Autodesk Fusion 360 part; units mm, degrees
(part 33 of 40)
  spline S112 degree 5 poles (166.3167, 190.3263) (166.2935, 190.3467) (166.2466, 190.3868) (166.1747, 190.4451) (166.076, 190.5192) (165.9487, 190.6066) (165.8185, 190.6904) (165.6866, 190.772) (165.5538, 190.8524) (165.4203, 190.932) (165.2862, 191.0107) (165.1513, 191.0883) (165.0152, 191.1642) (164.8777, 191.2383) (164.739, 191.3106) (164.5991, 191.3813) (164.4582, 191.4504) (164.3164, 191.5184) (164.1739, 191.5853) (164.0308, 191.6512) (163.887, 191.716) (163.7425, 191.7798) (163.5973, 191.8424) (163.4513, 191.9039) (163.3046, 191.9642) (163.1571, 192.0234) (163.009, 192.0815) (162.8603, 192.1386) (162.711, 192.1947) (162.5611, 192.2499) (162.4106, 192.3041) (162.2596, 192.3574) (162.108, 192.4097) (161.9559, 192.461) (161.8032, 192.5114) (161.65, 192.5608) (161.4962, 192.6094) (161.342, 192.657) (161.1873, 192.7037) (161.0321, 192.7495) (160.8764, 192.7945) (160.7202, 192.8386) (160.5636, 192.8818) (160.4065, 192.9241) (160.249, 192.9656) (160.0911, 193.0063) (159.9327, 193.0461) (159.7739, 193.085) (159.6147, 193.1231) (159.4551, 193.1604) (159.2951, 193.1969) (159.1347, 193.2326) (158.9739, 193.2674) (158.8127, 193.3015) (158.6511, 193.3347) (158.4892, 193.3672) (158.3269, 193.3988) (158.1643, 193.4297) (158.0013, 193.4597) (157.838, 193.489) (157.6743, 193.5175) (157.5103, 193.5453) (157.3459, 193.5723) (157.1812, 193.5984) (157.0162, 193.6239) (156.8509, 193.6486) (156.6853, 193.6725) (156.5194, 193.6956) (156.3531, 193.718) (156.1866, 193.7397) (156.0198, 193.7606) (155.8861, 193.7767) (155.7857, 193.7885) (155.7187, 193.7962) (155.6851, 193.8) knots 0 0 0 0 0 0 0.01428571 0.02857143 0.04285714 0.05714286 0.07142857 0.08571429 0.1 0.11428571 0.12857143 0.14285714 0.15714286 0.17142857 0.18571429 0.2 0.21428571 0.22857143 0.24285714 0.25714286 0.27142857 0.28571429 0.3 0.31428571 0.32857143 0.34285714 0.35714286 0.37142857 0.38571429 0.4 0.41428571 0.42857143 0.44285714 0.45714286 0.47142857 0.48571429 0.5 0.51428571 0.52857143 0.54285714 0.55714286 0.57142857 0.58571429 0.6 0.61428571 0.62857143 0.64285714 0.65714286 0.67142857 0.68571429 0.7 0.71428571 0.72857143 0.74285714 0.75714286 0.77142857 0.78571429 0.8 0.81428571 0.82857143 0.84285714 0.85714286 0.87142857 0.88571429 0.9 0.91428571 0.92857143 0.94285714 0.95714286 0.97142857 0.98571429 1 1 1 1 1 1
  line L8400 (166.3167, 190.3263) -> (166.2935, 190.3467) construction
  line L8401 (166.2935, 190.3467) -> (166.2466, 190.3868) construction
  line L8402 (166.2466, 190.3868) -> (166.1747, 190.4451) construction
  line L8403 (166.1747, 190.4451) -> (166.076, 190.5192) construction
  line L8404 (166.076, 190.5192) -> (165.9487, 190.6066) construction
  line L8405 (165.9487, 190.6066) -> (165.8185, 190.6904) construction
  line L8406 (165.8185, 190.6904) -> (165.6866, 190.772) construction
  line L8407 (165.6866, 190.772) -> (165.5538, 190.8524) construction
  line L8408 (165.5538, 190.8524) -> (165.4203, 190.932) construction
  line L8409 (165.4203, 190.932) -> (165.2862, 191.0107) construction
  line L8410 (165.2862, 191.0107) -> (165.1513, 191.0883) construction
  line L8411 (165.1513, 191.0883) -> (165.0152, 191.1642) construction
  line L8412 (165.0152, 191.1642) -> (164.8777, 191.2383) construction
  line L8413 (164.8777, 191.2383) -> (164.739, 191.3106) construction
  line L8414 (164.739, 191.3106) -> (164.5991, 191.3813) construction
  line L8415 (164.5991, 191.3813) -> (164.4582, 191.4504) construction
  line L8416 (164.4582, 191.4504) -> (164.3164, 191.5184) construction
  line L8417 (164.3164, 191.5184) -> (164.1739, 191.5853) construction
  line L8418 (164.1739, 191.5853) -> (164.0308, 191.6512) construction
  line L8419 (164.0308, 191.6512) -> (163.887, 191.716) construction
  line L8420 (163.887, 191.716) -> (163.7425, 191.7798) construction
  line L8421 (163.7425, 191.7798) -> (163.5973, 191.8424) construction
  line L8422 (163.5973, 191.8424) -> (163.4513, 191.9039) construction
  line L8423 (163.4513, 191.9039) -> (163.3046, 191.9642) construction
  line L8424 (163.3046, 191.9642) -> (163.1571, 192.0234) construction
  line L8425 (163.1571, 192.0234) -> (163.009, 192.0815) construction
  line L8426 (163.009, 192.0815) -> (162.8603, 192.1386) construction
  line L8427 (162.8603, 192.1386) -> (162.711, 192.1947) construction
  line L8428 (162.711, 192.1947) -> (162.5611, 192.2499) construction
  line L8429 (162.5611, 192.2499) -> (162.4106, 192.3041) construction
  line L8430 (162.4106, 192.3041) -> (162.2596, 192.3574) construction
  line L8431 (162.2596, 192.3574) -> (162.108, 192.4097) construction
  line L8432 (162.108, 192.4097) -> (161.9559, 192.461) construction
  line L8433 (161.9559, 192.461) -> (161.8032, 192.5114) construction
  line L8434 (161.8032, 192.5114) -> (161.65, 192.5608) construction
  line L8435 (161.65, 192.5608) -> (161.4962, 192.6094) construction
  line L8436 (161.4962, 192.6094) -> (161.342, 192.657) construction
  line L8437 (161.342, 192.657) -> (161.1873, 192.7037) construction
  line L8438 (161.1873, 192.7037) -> (161.0321, 192.7495) construction
  line L8439 (161.0321, 192.7495) -> (160.8764, 192.7945) construction
  line L8440 (160.8764, 192.7945) -> (160.7202, 192.8386) construction
  line L8441 (160.7202, 192.8386) -> (160.5636, 192.8818) construction
  line L8442 (160.5636, 192.8818) -> (160.4065, 192.9241) construction
  line L8443 (160.4065, 192.9241) -> (160.249, 192.9656) construction
  line L8444 (160.249, 192.9656) -> (160.0911, 193.0063) construction
  line L8445 (160.0911, 193.0063) -> (159.9327, 193.0461) construction
  line L8446 (159.9327, 193.0461) -> (159.7739, 193.085) construction
  line L8447 (159.7739, 193.085) -> (159.6147, 193.1231) construction
  line L8448 (159.6147, 193.1231) -> (159.4551, 193.1604) construction
  line L8449 (159.4551, 193.1604) -> (159.2951, 193.1969) construction
  line L8450 (159.2951, 193.1969) -> (159.1347, 193.2326) construction
  line L8451 (159.1347, 193.2326) -> (158.9739, 193.2674) construction
  line L8452 (158.9739, 193.2674) -> (158.8127, 193.3015) construction
  line L8453 (158.8127, 193.3015) -> (158.6511, 193.3347) construction
  line L8454 (158.6511, 193.3347) -> (158.4892, 193.3672) construction
  line L8455 (158.4892, 193.3672) -> (158.3269, 193.3988) construction
  line L8456 (158.3269, 193.3988) -> (158.1643, 193.4297) construction
  line L8457 (158.1643, 193.4297) -> (158.0013, 193.4597) construction
  line L8458 (158.0013, 193.4597) -> (157.838, 193.489) construction
  line L8459 (157.838, 193.489) -> (157.6743, 193.5175) construction
  line L8460 (157.6743, 193.5175) -> (157.5103, 193.5453) construction
  line L8461 (157.5103, 193.5453) -> (157.3459, 193.5723) construction
  line L8462 (157.3459, 193.5723) -> (157.1812, 193.5984) construction
  line L8463 (157.1812, 193.5984) -> (157.0162, 193.6239) construction
  line L8464 (157.0162, 193.6239) -> (156.8509, 193.6486) construction
  line L8465 (156.8509, 193.6486) -> (156.6853, 193.6725) construction
  line L8466 (156.6853, 193.6725) -> (156.5194, 193.6956) construction
  line L8467 (156.5194, 193.6956) -> (156.3531, 193.718) construction
  line L8468 (156.3531, 193.718) -> (156.1866, 193.7397) construction
  line L8469 (156.1866, 193.7397) -> (156.0198, 193.7606) construction
  line L8470 (156.0198, 193.7606) -> (155.8861, 193.7767) construction
  line L8471 (155.8861, 193.7767) -> (155.7857, 193.7885) construction
  line L8472 (155.7857, 193.7885) -> (155.7187, 193.7962) construction
  line L8473 (155.7187, 193.7962) -> (155.6851, 193.8) construction
  arc A209 (172.7536, 191.8132) -> (172.8837, 194.5906) centre (171.3824, 193.2692) ccw
  arc A210 (214.3883, 221.4115) -> (209.8757, 221.4115) centre (212.132, 150) ccw
  spline S113 degree 5 poles (166.3167, 109.6737) (166.2935, 109.6533) (166.2466, 109.6132) (166.1747, 109.5549) (166.076, 109.4808) (165.9487, 109.3934) (165.8185, 109.3096) (165.6866, 109.228) (165.5538, 109.1476) (165.4203, 109.068) (165.2862, 108.9893) (165.1513, 108.9117) (165.0152, 108.8358) (164.8777, 108.7617) (164.739, 108.6894) (164.5991, 108.6187) (164.4582, 108.5496) (164.3164, 108.4816) (164.1739, 108.4147) (164.0308, 108.3488) (163.887, 108.284) (163.7425, 108.2202) (163.5973, 108.1576) (163.4513, 108.0961) (163.3046, 108.0358) (163.1571, 107.9766) (163.009, 107.9185) (162.8603, 107.8614) (162.711, 107.8053) (162.5611, 107.7501) (162.4106, 107.6959) (162.2596, 107.6426) (162.108, 107.5903) (161.9559, 107.539) (161.8032, 107.4886) (161.65, 107.4392) (161.4962, 107.3906) (161.342, 107.343) (161.1873, 107.2963) (161.0321, 107.2505) (160.8764, 107.2055) (160.7202, 107.1614) (160.5636, 107.1182) (160.4065, 107.0759) (160.249, 107.0344) (160.0911, 106.9937) (159.9327, 106.9539) (159.7739, 106.915) (159.6147, 106.8769) (159.4551, 106.8396) (159.2951, 106.8031) (159.1347, 106.7674) (158.9739, 106.7326) (158.8127, 106.6985) (158.6511, 106.6653) (158.4892, 106.6328) (158.3269, 106.6012) (158.1643, 106.5703) (158.0013, 106.5403) (157.838, 106.511) (157.6743, 106.4825) (157.5103, 106.4547) (157.3459, 106.4277) (157.1812, 106.4016) (157.0162, 106.3761) (156.8509, 106.3514) (156.6853, 106.3275) (156.5194, 106.3044) (156.3531, 106.282) (156.1866, 106.2603) (156.0198, 106.2394) (155.8861, 106.2233) (155.7857, 106.2115) (155.7187, 106.2038) (155.6851, 106.2) knots 0 0 0 0 0 0 0.01428571 0.02857143 0.04285714 0.05714286 0.07142857 0.08571429 0.1 0.11428571 0.12857143 0.14285714 0.15714286 0.17142857 0.18571429 0.2 0.21428571 0.22857143 0.24285714 0.25714286 0.27142857 0.28571429 0.3 0.31428571 0.32857143 0.34285714 0.35714286 0.37142857 0.38571429 0.4 0.41428571 0.42857143 0.44285714 0.45714286 0.47142857 0.48571429 0.5 0.51428571 0.52857143 0.54285714 0.55714286 0.57142857 0.58571429 0.6 0.61428571 0.62857143 0.64285714 0.65714286 0.67142857 0.68571429 0.7 0.71428571 0.72857143 0.74285714 0.75714286 0.77142857 0.78571429 0.8 0.81428571 0.82857143 0.84285714 0.85714286 0.87142857 0.88571429 0.9 0.91428571 0.92857143 0.94285714 0.95714286 0.97142857 0.98571429 1 1 1 1 1 1
  line L8474 (166.3167, 109.6737) -> (166.2935, 109.6533) construction
  line L8475 (166.2935, 109.6533) -> (166.2466, 109.6132) construction
  line L8476 (166.2466, 109.6132) -> (166.1747, 109.5549) construction
  line L8477 (166.1747, 109.5549) -> (166.076, 109.4808) construction
  line L8478 (166.076, 109.4808) -> (165.9487, 109.3934) construction
  line L8479 (165.9487, 109.3934) -> (165.8185, 109.3096) construction
  line L8480 (165.8185, 109.3096) -> (165.6866, 109.228) construction
  line L8481 (165.6866, 109.228) -> (165.5538, 109.1476) construction
  line L8482 (165.5538, 109.1476) -> (165.4203, 109.068) construction
  line L8483 (165.4203, 109.068) -> (165.2862, 108.9893) construction
  line L8484 (165.2862, 108.9893) -> (165.1513, 108.9117) construction
  line L8485 (165.1513, 108.9117) -> (165.0152, 108.8358) construction
  line L8486 (165.0152, 108.8358) -> (164.8777, 108.7617) construction
  line L8487 (164.8777, 108.7617) -> (164.739, 108.6894) construction
  line L8488 (164.739, 108.6894) -> (164.5991, 108.6187) construction
  line L8489 (164.5991, 108.6187) -> (164.4582, 108.5496) construction
  line L8490 (164.4582, 108.5496) -> (164.3164, 108.4816) construction
  line L8491 (164.3164, 108.4816) -> (164.1739, 108.4147) construction
  line L8492 (164.1739, 108.4147) -> (164.0308, 108.3488) construction
  line L8493 (164.0308, 108.3488) -> (163.887, 108.284) construction
  line L8494 (163.887, 108.284) -> (163.7425, 108.2202) construction
  line L8495 (163.7425, 108.2202) -> (163.5973, 108.1576) construction
  line L8496 (163.5973, 108.1576) -> (163.4513, 108.0961) construction
  line L8497 (163.4513, 108.0961) -> (163.3046, 108.0358) construction
  line L8498 (163.3046, 108.0358) -> (163.1571, 107.9766) construction
  line L8499 (163.1571, 107.9766) -> (163.009, 107.9185) construction
  line L8500 (163.009, 107.9185) -> (162.8603, 107.8614) construction
  line L8501 (162.8603, 107.8614) -> (162.711, 107.8053) construction
  line L8502 (162.711, 107.8053) -> (162.5611, 107.7501) construction
  line L8503 (162.5611, 107.7501) -> (162.4106, 107.6959) construction
  line L8504 (162.4106, 107.6959) -> (162.2596, 107.6426) construction
  line L8505 (162.2596, 107.6426) -> (162.108, 107.5903) construction
  line L8506 (162.108, 107.5903) -> (161.9559, 107.539) construction
  line L8507 (161.9559, 107.539) -> (161.8032, 107.4886) construction
  line L8508 (161.8032, 107.4886) -> (161.65, 107.4392) construction
  line L8509 (161.65, 107.4392) -> (161.4962, 107.3906) construction
  line L8510 (161.4962, 107.3906) -> (161.342, 107.343) construction
  line L8511 (161.342, 107.343) -> (161.1873, 107.2963) construction
  line L8512 (161.1873, 107.2963) -> (161.0321, 107.2505) construction
  line L8513 (161.0321, 107.2505) -> (160.8764, 107.2055) construction
  line L8514 (160.8764, 107.2055) -> (160.7202, 107.1614) construction
  line L8515 (160.7202, 107.1614) -> (160.5636, 107.1182) construction
  line L8516 (160.5636, 107.1182) -> (160.4065, 107.0759) construction
  line L8517 (160.4065, 107.0759) -> (160.249, 107.0344) construction
  line L8518 (160.249, 107.0344) -> (160.0911, 106.9937) construction
  line L8519 (160.0911, 106.9937) -> (159.9327, 106.9539) construction
  line L8520 (159.9327, 106.9539) -> (159.7739, 106.915) construction
  line L8521 (159.7739, 106.915) -> (159.6147, 106.8769) construction
  line L8522 (159.6147, 106.8769) -> (159.4551, 106.8396) construction
  line L8523 (159.4551, 106.8396) -> (159.2951, 106.8031) construction
  line L8524 (159.2951, 106.8031) -> (159.1347, 106.7674) construction
  line L8525 (159.1347, 106.7674) -> (158.9739, 106.7326) construction
  line L8526 (158.9739, 106.7326) -> (158.8127, 106.6985) construction
  line L8527 (158.8127, 106.6985) -> (158.6511, 106.6653) construction
  line L8528 (158.6511, 106.6653) -> (158.4892, 106.6328) construction
  line L8529 (158.4892, 106.6328) -> (158.3269, 106.6012) construction
  line L8530 (158.3269, 106.6012) -> (158.1643, 106.5703) construction
  line L8531 (158.1643, 106.5703) -> (158.0013, 106.5403) construction
  line L8532 (158.0013, 106.5403) -> (157.838, 106.511) construction
  line L8533 (157.838, 106.511) -> (157.6743, 106.4825) construction
  line L8534 (157.6743, 106.4825) -> (157.5103, 106.4547) construction
  line L8535 (157.5103, 106.4547) -> (157.3459, 106.4277) construction
  line L8536 (157.3459, 106.4277) -> (157.1812, 106.4016) construction
  line L8537 (157.1812, 106.4016) -> (157.0162, 106.3761) construction
  line L8538 (157.0162, 106.3761) -> (156.8509, 106.3514) construction
  line L8539 (156.8509, 106.3514) -> (156.6853, 106.3275) construction
  line L8540 (156.6853, 106.3275) -> (156.5194, 106.3044) construction
  line L8541 (156.5194, 106.3044) -> (156.3531, 106.282) construction
  line L8542 (156.3531, 106.282) -> (156.1866, 106.2603) construction
  line L8543 (156.1866, 106.2603) -> (156.0198, 106.2394) construction
  line L8544 (156.0198, 106.2394) -> (155.8861, 106.2233) construction
  line L8545 (155.8861, 106.2233) -> (155.7857, 106.2115) construction
  line L8546 (155.7857, 106.2115) -> (155.7187, 106.2038) construction
  line L8547 (155.7187, 106.2038) -> (155.6851, 106.2) construction
  arc A211 (187.9188, 82.7809) -> (192.2105, 81.3864) centre (212.132, 150) ccw
  arc A212 (251.5104, 108.1868) -> (253.9452, 110.6216) centre (212.132, 150) ccw
  arc A213 (262.5041, 122.4018) -> (264.0674, 125.4699) centre (212.132, 150) ccw
  line L8548 (172.8837, 105.4094) -> (171.8057, 104.1847)
  line L8549 (199.127, 92.0377) -> (198.7698, 90.4458)
  line L8550 (235.6801, 95.4634) -> (236.3268, 93.9655)
  line L8551 (225.137, 92.0377) -> (225.4942, 90.4458)
  arc A214 (253.9452, 189.3784) -> (256.7226, 189.2483) centre (255.4012, 190.7496) ccw
  arc A215 (217.6748, 209.1442) -> (219.4126, 206.9737) centre (219.6661, 208.9575) ccw
  line L8552 (256.7226, 189.2483) -> (257.9473, 190.3263)
  line L8553 (161.0254, 119.7202) -> (159.6217, 118.8885)
  line L8554 (256.7226, 189.2483) -> (257.9473, 190.3263)
  line L8555 (270.0943, 163.005) -> (271.6862, 163.3622)
  line L8556 (271.2762, 144.4572) -> (272.9005, 144.3049)
  line L8557 (167.5414, 110.7517) -> (166.3167, 109.6737)
  arc A216 (252.2812, 90.9007) -> (255.932, 93.5531) centre (212.132, 150) ccw
  spline S114 degree 5 poles (268.1665, 174.1948) (268.1948, 174.2071) (268.2518, 174.2308) (268.3382, 174.264) (268.4549, 174.3039) (268.6031, 174.3478) (268.7528, 174.3873) (268.9034, 174.4241) (269.0546, 174.4595) (269.2061, 174.494) (269.358, 174.5274) (269.5103, 174.5594) (269.6632, 174.5896) (269.8168, 174.6176) (269.9711, 174.6435) (270.126, 174.6674) (270.2814, 174.6897) (270.4372, 174.7105) (270.5934, 174.7301) (270.7499, 174.7485) (270.9067, 174.7658) (271.0638, 174.7818) (271.2213, 174.7965) (271.3791, 174.8098) (271.5373, 174.8218) (271.6958, 174.8325) (271.8546, 174.842) (272.0137, 174.8504) (272.1731, 174.8577) (272.3327, 174.8638) (272.4925, 174.8689) (272.6526, 174.8729) (272.8129, 174.8757) (272.9735, 174.8776) (273.1343, 174.8783) (273.2953, 174.878) (273.4565, 174.8766) (273.6179, 174.8742) (273.7795, 174.8708) (273.9413, 174.8665) (274.1032, 174.8611) (274.2654, 174.8548) (274.4277, 174.8475) (274.5901, 174.8392) (274.7527, 174.83) (274.9155, 174.8199) (275.0784, 174.8088) (275.2415, 174.7967) (275.4047, 174.7838) (275.568, 174.77) (275.7315, 174.7552) (275.8951, 174.7396) (276.0588, 174.723) (276.2226, 174.7056) (276.3865, 174.6873) (276.5505, 174.6681) (276.7146, 174.648) (276.8788, 174.6271) (277.0431, 174.6054) (277.2075, 174.5828) (277.372, 174.5593) (277.5366, 174.535) (277.7012, 174.5098) (277.866, 174.4839) (278.0307, 174.4571) (278.1956, 174.4294) (278.3605, 174.401) (278.5255, 174.3718) (278.6905, 174.3417) (278.8556, 174.3108) (279.0207, 174.2792) (279.1528, 174.2532) (279.2519, 174.2334) (279.318, 174.22) (279.3511, 174.2132) knots 0 0 0 0 0 0 0.01428571 0.02857143 0.04285714 0.05714286 0.07142857 0.08571429 0.1 0.11428571 0.12857143 0.14285714 0.15714286 0.17142857 0.18571429 0.2 0.21428571 0.22857143 0.24285714 0.25714286 0.27142857 0.28571429 0.3 0.31428571 0.32857143 0.34285714 0.35714286 0.37142857 0.38571429 0.4 0.41428571 0.42857143 0.44285714 0.45714286 0.47142857 0.48571429 0.5 0.51428571 0.52857143 0.54285714 0.55714286 0.57142857 0.58571429 0.6 0.61428571 0.62857143 0.64285714 0.65714286 0.67142857 0.68571429 0.7 0.71428571 0.72857143 0.74285714 0.75714286 0.77142857 0.78571429 0.8 0.81428571 0.82857143 0.84285714 0.85714286 0.87142857 0.88571429 0.9 0.91428571 0.92857143 0.94285714 0.95714286 0.97142857 0.98571429 1 1 1 1 1 1
  line L8558 (268.1665, 174.1948) -> (268.1948, 174.2071) construction
  line L8559 (268.1948, 174.2071) -> (268.2518, 174.2308) construction
  line L8560 (268.2518, 174.2308) -> (268.3382, 174.264) construction
  line L8561 (268.3382, 174.264) -> (268.4549, 174.3039) construction
  line L8562 (268.4549, 174.3039) -> (268.6031, 174.3478) construction
  line L8563 (268.6031, 174.3478) -> (268.7528, 174.3873) construction
  line L8564 (268.7528, 174.3873) -> (268.9034, 174.4241) construction
  line L8565 (268.9034, 174.4241) -> (269.0546, 174.4595) construction
  line L8566 (269.0546, 174.4595) -> (269.2061, 174.494) construction
  line L8567 (269.2061, 174.494) -> (269.358, 174.5274) construction
  line L8568 (269.358, 174.5274) -> (269.5103, 174.5594) construction
  line L8569 (269.5103, 174.5594) -> (269.6632, 174.5896) construction
  line L8570 (269.6632, 174.5896) -> (269.8168, 174.6176) construction
  line L8571 (269.8168, 174.6176) -> (269.9711, 174.6435) construction
  line L8572 (269.9711, 174.6435) -> (270.126, 174.6674) construction
  line L8573 (270.126, 174.6674) -> (270.2814, 174.6897) construction
  line L8574 (270.2814, 174.6897) -> (270.4372, 174.7105) construction
  line L8575 (270.4372, 174.7105) -> (270.5934, 174.7301) construction
  line L8576 (270.5934, 174.7301) -> (270.7499, 174.7485) construction
  line L8577 (270.7499, 174.7485) -> (270.9067, 174.7658) construction
  line L8578 (270.9067, 174.7658) -> (271.0638, 174.7818) construction
  line L8579 (271.0638, 174.7818) -> (271.2213, 174.7965) construction
  line L8580 (271.2213, 174.7965) -> (271.3791, 174.8098) construction
  line L8581 (271.3791, 174.8098) -> (271.5373, 174.8218) construction
  line L8582 (271.5373, 174.8218) -> (271.6958, 174.8325) construction
  line L8583 (271.6958, 174.8325) -> (271.8546, 174.842) construction
  line L8584 (271.8546, 174.842) -> (272.0137, 174.8504) construction
  line L8585 (272.0137, 174.8504) -> (272.1731, 174.8577) construction
  line L8586 (272.1731, 174.8577) -> (272.3327, 174.8638) construction
  line L8587 (272.3327, 174.8638) -> (272.4925, 174.8689) construction
  line L8588 (272.4925, 174.8689) -> (272.6526, 174.8729) construction
  line L8589 (272.6526, 174.8729) -> (272.8129, 174.8757) construction
  line L8590 (272.8129, 174.8757) -> (272.9735, 174.8776) construction
  line L8591 (272.9735, 174.8776) -> (273.1343, 174.8783) construction
  line L8592 (273.1343, 174.8783) -> (273.2953, 174.878) construction
  line L8593 (273.2953, 174.878) -> (273.4565, 174.8766) construction
  line L8594 (273.4565, 174.8766) -> (273.6179, 174.8742) construction
  line L8595 (273.6179, 174.8742) -> (273.7795, 174.8708) construction
  line L8596 (273.7795, 174.8708) -> (273.9413, 174.8665) construction
  line L8597 (273.9413, 174.8665) -> (274.1032, 174.8611) construction
  line L8598 (274.1032, 174.8611) -> (274.2654, 174.8548) construction
  line L8599 (274.2654, 174.8548) -> (274.4277, 174.8475) construction
  line L8600 (274.4277, 174.8475) -> (274.5901, 174.8392) construction
  line L8601 (274.5901, 174.8392) -> (274.7527, 174.83) construction
  line L8602 (274.7527, 174.83) -> (274.9155, 174.8199) construction
  line L8603 (274.9155, 174.8199) -> (275.0784, 174.8088) construction
  line L8604 (275.0784, 174.8088) -> (275.2415, 174.7967) construction
  line L8605 (275.2415, 174.7967) -> (275.4047, 174.7838) construction
  line L8606 (275.4047, 174.7838) -> (275.568, 174.77) construction
  line L8607 (275.568, 174.77) -> (275.7315, 174.7552) construction
  line L8608 (275.7315, 174.7552) -> (275.8951, 174.7396) construction
  line L8609 (275.8951, 174.7396) -> (276.0588, 174.723) construction
  line L8610 (276.0588, 174.723) -> (276.2226, 174.7056) construction
  line L8611 (276.2226, 174.7056) -> (276.3865, 174.6873) construction
  line L8612 (276.3865, 174.6873) -> (276.5505, 174.6681) construction
  line L8613 (276.5505, 174.6681) -> (276.7146, 174.648) construction
  line L8614 (276.7146, 174.648) -> (276.8788, 174.6271) construction
  line L8615 (276.8788, 174.6271) -> (277.0431, 174.6054) construction
  line L8616 (277.0431, 174.6054) -> (277.2075, 174.5828) construction
  line L8617 (277.2075, 174.5828) -> (277.372, 174.5593) construction
  line L8618 (277.372, 174.5593) -> (277.5366, 174.535) construction
  line L8619 (277.5366, 174.535) -> (277.7012, 174.5098) construction
  line L8620 (277.7012, 174.5098) -> (277.866, 174.4839) construction
  line L8621 (277.866, 174.4839) -> (278.0307, 174.4571) construction
  line L8622 (278.0307, 174.4571) -> (278.1956, 174.4294) construction
  line L8623 (278.1956, 174.4294) -> (278.3605, 174.401) construction
  line L8624 (278.3605, 174.401) -> (278.5255, 174.3718) construction
  line L8625 (278.5255, 174.3718) -> (278.6905, 174.3417) construction
  line L8626 (278.6905, 174.3417) -> (278.8556, 174.3108) construction
  line L8627 (278.8556, 174.3108) -> (279.0207, 174.2792) construction
  line L8628 (279.0207, 174.2792) -> (279.1528, 174.2532) construction
  line L8629 (279.1528, 174.2532) -> (279.2519, 174.2334) construction
  line L8630 (279.2519, 174.2334) -> (279.318, 174.22) construction
  line L8631 (279.318, 174.22) -> (279.3511, 174.2132) construction
  arc A217 (209.8757, 78.5885) -> (214.3883, 78.5885) centre (212.132, 150) ccw
  spline S115 degree 5 poles (198.7698, 209.5542) (198.763, 209.5843) (198.7487, 209.6444) (198.7249, 209.7338) (198.6885, 209.8517) (198.6369, 209.9973) (198.5809, 210.1416) (198.5221, 210.2852) (198.4619, 210.4283) (198.4007, 210.5711) (198.3385, 210.7136) (198.2749, 210.8557) (198.2094, 210.9971) (198.1418, 211.1379) (198.072, 211.2779) (198.0004, 211.4173) (197.927, 211.5561) (197.8523, 211.6944) (197.7763, 211.8322) (197.6993, 211.9697) (197.6211, 212.1067) (197.5416, 212.2432) (197.4609, 212.3792) (197.379, 212.5148) (197.2957, 212.6498) (197.2112, 212.7843) (197.1256, 212.9184) (197.0388, 213.052) (196.951, 213.1852) (196.8622, 213.318) (196.7723, 213.4503) (196.6814, 213.5821) (196.5895, 213.7135) (196.4966, 213.8445) (196.4027, 213.975) (196.3078, 214.105) (196.212, 214.2346) (196.1152, 214.3638) (196.0174, 214.4926) (195.9188, 214.6209) (195.8193, 214.7488) (195.7189, 214.8762) (195.6176, 215.0032) (195.5154, 215.1298) (195.4124, 215.256) (195.3085, 215.3817) (195.2037, 215.507) (195.0982, 215.6318) (194.9918, 215.7562) (194.8846, 215.8802) (194.7765, 216.0038) (194.6677, 216.1269) (194.5581, 216.2497) (194.4478, 216.3719) (194.3366, 216.4938) (194.2247, 216.6152) (194.112, 216.7362) (193.9985, 216.8568) (193.8843, 216.9769) (193.7694, 217.0966) (193.6538, 217.2159) (193.5374, 217.3347) (193.4202, 217.4531) (193.3024, 217.5711) (193.1839, 217.6887) (193.0646, 217.8058) (192.9447, 217.9225) (192.8241, 218.0388) (192.7027, 218.1546) (192.5808, 218.27) (192.4581, 218.385) (192.3594, 218.4767) (192.2851, 218.5452) (192.2354, 218.5908) (192.2105, 218.6136) knots 0 0 0 0 0 0 0.01428571 0.02857143 0.04285714 0.05714286 0.07142857 0.08571429 0.1 0.11428571 0.12857143 0.14285714 0.15714286 0.17142857 0.18571429 0.2 0.21428571 0.22857143 0.24285714 0.25714286 0.27142857 0.28571429 0.3 0.31428571 0.32857143 0.34285714 0.35714286 0.37142857 0.38571429 0.4 0.41428571 0.42857143 0.44285714 0.45714286 0.47142857 0.48571429 0.5 0.51428571 0.52857143 0.54285714 0.55714286 0.57142857 0.58571429 0.6 0.61428571 0.62857143 0.64285714 0.65714286 0.67142857 0.68571429 0.7 0.71428571 0.72857143 0.74285714 0.75714286 0.77142857 0.78571429 0.8 0.81428571 0.82857143 0.84285714 0.85714286 0.87142857 0.88571429 0.9 0.91428571 0.92857143 0.94285714 0.95714286 0.97142857 0.98571429 1 1 1 1 1 1
  line L8632 (198.7698, 209.5542) -> (198.763, 209.5843) construction
  line L8633 (198.763, 209.5843) -> (198.7487, 209.6444) construction
  line L8634 (198.7487, 209.6444) -> (198.7249, 209.7338) construction
  line L8635 (198.7249, 209.7338) -> (198.6885, 209.8517) construction
  line L8636 (198.6885, 209.8517) -> (198.6369, 209.9973) construction
  line L8637 (198.6369, 209.9973) -> (198.5809, 210.1416) construction
  line L8638 (198.5809, 210.1416) -> (198.5221, 210.2852) construction
  line L8639 (198.5221, 210.2852) -> (198.4619, 210.4283) construction
  line L8640 (198.4619, 210.4283) -> (198.4007, 210.5711) construction
  line L8641 (198.4007, 210.5711) -> (198.3385, 210.7136) construction
  line L8642 (198.3385, 210.7136) -> (198.2749, 210.8557) construction
  line L8643 (198.2749, 210.8557) -> (198.2094, 210.9971) construction
  line L8644 (198.2094, 210.9971) -> (198.1418, 211.1379) construction
  line L8645 (198.1418, 211.1379) -> (198.072, 211.2779) construction
  line L8646 (198.072, 211.2779) -> (198.0004, 211.4173) construction
  line L8647 (198.0004, 211.4173) -> (197.927, 211.5561) construction
  line L8648 (197.927, 211.5561) -> (197.8523, 211.6944) construction
  line L8649 (197.8523, 211.6944) -> (197.7763, 211.8322) construction
  line L8650 (197.7763, 211.8322) -> (197.6993, 211.9697) construction
  line L8651 (197.6993, 211.9697) -> (197.6211, 212.1067) construction
  line L8652 (197.6211, 212.1067) -> (197.5416, 212.2432) construction
  line L8653 (197.5416, 212.2432) -> (197.4609, 212.3792) construction
  line L8654 (197.4609, 212.3792) -> (197.379, 212.5148) construction
  line L8655 (197.379, 212.5148) -> (197.2957, 212.6498) construction
  line L8656 (197.2957, 212.6498) -> (197.2112, 212.7843) construction
  line L8657 (197.2112, 212.7843) -> (197.1256, 212.9184) construction
  line L8658 (197.1256, 212.9184) -> (197.0388, 213.052) construction
  line L8659 (197.0388, 213.052) -> (196.951, 213.1852) construction
  line L8660 (196.951, 213.1852) -> (196.8622, 213.318) construction
  line L8661 (196.8622, 213.318) -> (196.7723, 213.4503) construction
  line L8662 (196.7723, 213.4503) -> (196.6814, 213.5821) construction
  line L8663 (196.6814, 213.5821) -> (196.5895, 213.7135) construction
  line L8664 (196.5895, 213.7135) -> (196.4966, 213.8445) construction
  line L8665 (196.4966, 213.8445) -> (196.4027, 213.975) construction
  line L8666 (196.4027, 213.975) -> (196.3078, 214.105) construction
  line L8667 (196.3078, 214.105) -> (196.212, 214.2346) construction
  line L8668 (196.212, 214.2346) -> (196.1152, 214.3638) construction
  line L8669 (196.1152, 214.3638) -> (196.0174, 214.4926) construction
  line L8670 (196.0174, 214.4926) -> (195.9188, 214.6209) construction
  line L8671 (195.9188, 214.6209) -> (195.8193, 214.7488) construction
  line L8672 (195.8193, 214.7488) -> (195.7189, 214.8762) construction
  line L8673 (195.7189, 214.8762) -> (195.6176, 215.0032) construction
  line L8674 (195.6176, 215.0032) -> (195.5154, 215.1298) construction
  line L8675 (195.5154, 215.1298) -> (195.4124, 215.256) construction
  line L8676 (195.4124, 215.256) -> (195.3085, 215.3817) construction
  line L8677 (195.3085, 215.3817) -> (195.2037, 215.507) construction
  line L8678 (195.2037, 215.507) -> (195.0982, 215.6318) construction
  line L8679 (195.0982, 215.6318) -> (194.9918, 215.7562) construction
  line L8680 (194.9918, 215.7562) -> (194.8846, 215.8802) construction
  line L8681 (194.8846, 215.8802) -> (194.7765, 216.0038) construction
  line L8682 (194.7765, 216.0038) -> (194.6677, 216.1269) construction
  line L8683 (194.6677, 216.1269) -> (194.5581, 216.2497) construction
  line L8684 (194.5581, 216.2497) -> (194.4478, 216.3719) construction
  line L8685 (194.4478, 216.3719) -> (194.3366, 216.4938) construction
  line L8686 (194.3366, 216.4938) -> (194.2247, 216.6152) construction
  line L8687 (194.2247, 216.6152) -> (194.112, 216.7362) construction
  line L8688 (194.112, 216.7362) -> (193.9985, 216.8568) construction
  line L8689 (193.9985, 216.8568) -> (193.8843, 216.9769) construction
  line L8690 (193.8843, 216.9769) -> (193.7694, 217.0966) construction
  line L8691 (193.7694, 217.0966) -> (193.6538, 217.2159) construction
  line L8692 (193.6538, 217.2159) -> (193.5374, 217.3347) construction
  line L8693 (193.5374, 217.3347) -> (193.4202, 217.4531) construction
  line L8694 (193.4202, 217.4531) -> (193.3024, 217.5711) construction
  line L8695 (193.3024, 217.5711) -> (193.1839, 217.6887) construction
  line L8696 (193.1839, 217.6887) -> (193.0646, 217.8058) construction
  line L8697 (193.0646, 217.8058) -> (192.9447, 217.9225) construction
  line L8698 (192.9447, 217.9225) -> (192.8241, 218.0388) construction
  line L8699 (192.8241, 218.0388) -> (192.7027, 218.1546) construction
  line L8700 (192.7027, 218.1546) -> (192.5808, 218.27) construction
  line L8701 (192.5808, 218.27) -> (192.4581, 218.385) construction
  line L8702 (192.4581, 218.385) -> (192.3594, 218.4767) construction
  line L8703 (192.3594, 218.4767) -> (192.2851, 218.5452) construction
  line L8704 (192.2851, 218.5452) -> (192.2354, 218.5908) construction
  line L8705 (192.2354, 218.5908) -> (192.2105, 218.6136) construction
  arc A218 (251.3803, 194.5906) -> (251.5104, 191.8132) centre (252.8816, 193.2692) ccw
  spline S116 degree 5 poles (264.6423, 118.8885) (264.6688, 118.8728) (264.7215, 118.8406) (264.7992, 118.7903) (264.9001, 118.7193) (265.0226, 118.6252) (265.1426, 118.5273) (265.2609, 118.4271) (265.3784, 118.3256) (265.4954, 118.2233) (265.6117, 118.12) (265.7271, 118.0156) (265.8414, 117.9097) (265.9544, 117.8019) (266.066, 117.6923) (266.1764, 117.581) (266.2857, 117.4684) (266.3942, 117.3545) (266.5018, 117.2397) (266.6087, 117.124) (266.7148, 117.0073) (266.8201, 116.8895) (266.9246, 116.7708) (267.0281, 116.6509) (267.1308, 116.53) (267.2327, 116.4081) (267.3337, 116.2852) (267.434, 116.1614) (267.5335, 116.0367) (267.6323, 115.9112) (267.7304, 115.7849) (267.8277, 115.6577) (267.9243, 115.5297) (268.0201, 115.4009) (268.1152, 115.2712) (268.2096, 115.1408) (268.3032, 115.0095) (268.3962, 114.8776) (268.4884, 114.7448) (268.58, 114.6114) (268.6708, 114.4772) (268.761, 114.3423) (268.8505, 114.2067) (268.9393, 114.0705) (269.0275, 113.9335) (269.1149, 113.7958) (269.2017, 113.6575) (269.2878, 113.5185) (269.3733, 113.3789) (269.4581, 113.2386) (269.5422, 113.0977) (269.6257, 112.9562) (269.7085, 112.814) (269.7907, 112.6712) (269.8723, 112.5279) (269.9532, 112.3839) (270.0334, 112.2393) (270.113, 112.0942) (270.192, 111.9485) (270.2703, 111.8022) (270.348, 111.6553) (270.4251, 111.5079) (270.5015, 111.3599) (270.5773, 111.2114) (270.6525, 111.0623) (270.727, 110.9127) (270.801, 110.7626) (270.8743, 110.6119) (270.9469, 110.4607) (271.019, 110.3091) (271.0904, 110.1569) (271.1471, 110.0347) (271.1893, 109.9428) (271.2173, 109.8815) (271.2313, 109.8508) knots 0 0 0 0 0 0 0.01428571 0.02857143 0.04285714 0.05714286 0.07142857 0.08571429 0.1 0.11428571 0.12857143 0.14285714 0.15714286 0.17142857 0.18571429 0.2 0.21428571 0.22857143 0.24285714 0.25714286 0.27142857 0.28571429 0.3 0.31428571 0.32857143 0.34285714 0.35714286 0.37142857 0.38571429 0.4 0.41428571 0.42857143 0.44285714 0.45714286 0.47142857 0.48571429 0.5 0.51428571 0.52857143 0.54285714 0.55714286 0.57142857 0.58571429 0.6 0.61428571 0.62857143 0.64285714 0.65714286 0.67142857 0.68571429 0.7 0.71428571 0.72857143 0.74285714 0.75714286 0.77142857 0.78571429 0.8 0.81428571 0.82857143 0.84285714 0.85714286 0.87142857 0.88571429 0.9 0.91428571 0.92857143 0.94285714 0.95714286 0.97142857 0.98571429 1 1 1 1 1 1
  line L8706 (264.6423, 118.8885) -> (264.6688, 118.8728) construction
  line L8707 (264.6688, 118.8728) -> (264.7215, 118.8406) construction
  line L8708 (264.7215, 118.8406) -> (264.7992, 118.7903) construction
  line L8709 (264.7992, 118.7903) -> (264.9001, 118.7193) construction
  line L8710 (264.9001, 118.7193) -> (265.0226, 118.6252) construction
  line L8711 (265.0226, 118.6252) -> (265.1426, 118.5273) construction
  line L8712 (265.1426, 118.5273) -> (265.2609, 118.4271) construction
  line L8713 (265.2609, 118.4271) -> (265.3784, 118.3256) construction
  line L8714 (265.3784, 118.3256) -> (265.4954, 118.2233) construction
  line L8715 (265.4954, 118.2233) -> (265.6117, 118.12) construction
  line L8716 (265.6117, 118.12) -> (265.7271, 118.0156) construction
  line L8717 (265.7271, 118.0156) -> (265.8414, 117.9097) construction
  line L8718 (265.8414, 117.9097) -> (265.9544, 117.8019) construction
  line L8719 (265.9544, 117.8019) -> (266.066, 117.6923) construction
  line L8720 (266.066, 117.6923) -> (266.1764, 117.581) construction
  line L8721 (266.1764, 117.581) -> (266.2857, 117.4684) construction
  line L8722 (266.2857, 117.4684) -> (266.3942, 117.3545) construction
  line L8723 (266.3942, 117.3545) -> (266.5018, 117.2397) construction
  line L8724 (266.5018, 117.2397) -> (266.6087, 117.124) construction
  line L8725 (266.6087, 117.124) -> (266.7148, 117.0073) construction
  line L8726 (266.7148, 117.0073) -> (266.8201, 116.8895) construction
  line L8727 (266.8201, 116.8895) -> (266.9246, 116.7708) construction
  line L8728 (266.9246, 116.7708) -> (267.0281, 116.6509) construction
  line L8729 (267.0281, 116.6509) -> (267.1308, 116.53) construction
  line L8730 (267.1308, 116.53) -> (267.2327, 116.4081) construction
  line L8731 (267.2327, 116.4081) -> (267.3337, 116.2852) construction
  line L8732 (267.3337, 116.2852) -> (267.434, 116.1614) construction
  line L8733 (267.434, 116.1614) -> (267.5335, 116.0367) construction
  line L8734 (267.5335, 116.0367) -> (267.6323, 115.9112) construction
  line L8735 (267.6323, 115.9112) -> (267.7304, 115.7849) construction
  line L8736 (267.7304, 115.7849) -> (267.8277, 115.6577) construction
  line L8737 (267.8277, 115.6577) -> (267.9243, 115.5297) construction
  line L8738 (267.9243, 115.5297) -> (268.0201, 115.4009) construction
  line L8739 (268.0201, 115.4009) -> (268.1152, 115.2712) construction
  line L8740 (268.1152, 115.2712) -> (268.2096, 115.1408) construction
  line L8741 (268.2096, 115.1408) -> (268.3032, 115.0095) construction
  line L8742 (268.3032, 115.0095) -> (268.3962, 114.8776) construction
  line L8743 (268.3962, 114.8776) -> (268.4884, 114.7448) construction
  line L8744 (268.4884, 114.7448) -> (268.58, 114.6114) construction
  line L8745 (268.58, 114.6114) -> (268.6708, 114.4772) construction
  line L8746 (268.6708, 114.4772) -> (268.761, 114.3423) construction
  line L8747 (268.761, 114.3423) -> (268.8505, 114.2067) construction
  line L8748 (268.8505, 114.2067) -> (268.9393, 114.0705) construction
  line L8749 (268.9393, 114.0705) -> (269.0275, 113.9335) construction
  line L8750 (269.0275, 113.9335) -> (269.1149, 113.7958) construction
  line L8751 (269.1149, 113.7958) -> (269.2017, 113.6575) construction
  line L8752 (269.2017, 113.6575) -> (269.2878, 113.5185) construction
  line L8753 (269.2878, 113.5185) -> (269.3733, 113.3789) construction
  line L8754 (269.3733, 113.3789) -> (269.4581, 113.2386) construction
  line L8755 (269.4581, 113.2386) -> (269.5422, 113.0977) construction
  line L8756 (269.5422, 113.0977) -> (269.6257, 112.9562) construction
  line L8757 (269.6257, 112.9562) -> (269.7085, 112.814) construction
  line L8758 (269.7085, 112.814) -> (269.7907, 112.6712) construction
  line L8759 (269.7907, 112.6712) -> (269.8723, 112.5279) construction
  line L8760 (269.8723, 112.5279) -> (269.9532, 112.3839) construction
  line L8761 (269.9532, 112.3839) -> (270.0334, 112.2393) construction
  line L8762 (270.0334, 112.2393) -> (270.113, 112.0942) construction
  line L8763 (270.113, 112.0942) -> (270.192, 111.9485) construction
  line L8764 (270.192, 111.9485) -> (270.2703, 111.8022) construction
  line L8765 (270.2703, 111.8022) -> (270.348, 111.6553) construction
  line L8766 (270.348, 111.6553) -> (270.4251, 111.5079) construction
  line L8767 (270.4251, 111.5079) -> (270.5015, 111.3599) construction
  line L8768 (270.5015, 111.3599) -> (270.5773, 111.2114) construction
  line L8769 (270.5773, 111.2114) -> (270.6525, 111.0623) construction
  line L8770 (270.6525, 111.0623) -> (270.727, 110.9127) construction
  line L8771 (270.727, 110.9127) -> (270.801, 110.7626) construction
  line L8772 (270.801, 110.7626) -> (270.8743, 110.6119) construction
  line L8773 (270.8743, 110.6119) -> (270.9469, 110.4607) construction
  line L8774 (270.9469, 110.4607) -> (271.019, 110.3091) construction
  line L8775 (271.019, 110.3091) -> (271.0904, 110.1569) construction
  line L8776 (271.0904, 110.1569) -> (271.1471, 110.0347) construction
  line L8777 (271.1471, 110.0347) -> (271.1893, 109.9428) construction
  line L8778 (271.1893, 109.9428) -> (271.2173, 109.8815) construction
  line L8779 (271.2173, 109.8815) -> (271.2313, 109.8508) construction
  spline S117 degree 5 poles (271.6862, 163.3622) (271.7163, 163.369) (271.7764, 163.3833) (271.8658, 163.4071) (271.9837, 163.4435) (272.1293, 163.4951) (272.2736, 163.5511) (272.4172, 163.6099) (272.5603, 163.6701) (272.7031, 163.7313) (272.8456, 163.7935) (272.9877, 163.8571) (273.1291, 163.9226) (273.2699, 163.9902) (273.4099, 164.06) (273.5493, 164.1316) (273.6881, 164.205) (273.8264, 164.2797) (273.9642, 164.3557) (274.1017, 164.4327) (274.2387, 164.5109) (274.3752, 164.5904) (274.5112, 164.6711) (274.6468, 164.753) (274.7818, 164.8363) (274.9163, 164.9208) (275.0504, 165.0064) (275.184, 165.0932) (275.3172, 165.181) (275.45, 165.2698) (275.5823, 165.3597) (275.7141, 165.4506) (275.8455, 165.5425) (275.9765, 165.6354) (276.107, 165.7293) (276.237, 165.8242) (276.3666, 165.92) (276.4958, 166.0168) (276.6246, 166.1146) (276.7529, 166.2132) (276.8808, 166.3127) (277.0082, 166.4131) (277.1352, 166.5144) (277.2618, 166.6166) (277.388, 166.7196) (277.5137, 166.8235) (277.639, 166.9283) (277.7638, 167.0338) (277.8882, 167.1402) (278.0122, 167.2474) (278.1358, 167.3555) (278.2589, 167.4643) (278.3817, 167.5739) (278.5039, 167.6842) (278.6258, 167.7954) (278.7472, 167.9073) (278.8682, 168.02) (278.9888, 168.1335) (279.1089, 168.2477) (279.2286, 168.3626) (279.3479, 168.4782) (279.4667, 168.5946) (279.5851, 168.7118) (279.7031, 168.8296) (279.8207, 168.9481) (279.9378, 169.0674) (280.0545, 169.1873) (280.1708, 169.3079) (280.2866, 169.4293) (280.402, 169.5512) (280.517, 169.6739) (280.6087, 169.7726) (280.6772, 169.8469) (280.7228, 169.8966) (280.7456, 169.9215) knots 0 0 0 0 0 0 0.01428571 0.02857143 0.04285714 0.05714286 0.07142857 0.08571429 0.1 0.11428571 0.12857143 0.14285714 0.15714286 0.17142857 0.18571429 0.2 0.21428571 0.22857143 0.24285714 0.25714286 0.27142857 0.28571429 0.3 0.31428571 0.32857143 0.34285714 0.35714286 0.37142857 0.38571429 0.4 0.41428571 0.42857143 0.44285714 0.45714286 0.47142857 0.48571429 0.5 0.51428571 0.52857143 0.54285714 0.55714286 0.57142857 0.58571429 0.6 0.61428571 0.62857143 0.64285714 0.65714286 0.67142857 0.68571429 0.7 0.71428571 0.72857143 0.74285714 0.75714286 0.77142857 0.78571429 0.8 0.81428571 0.82857143 0.84285714 0.85714286 0.87142857 0.88571429 0.9 0.91428571 0.92857143 0.94285714 0.95714286 0.97142857 0.98571429 1 1 1 1 1 1
  line L8780 (271.6862, 163.3622) -> (271.7163, 163.369) construction
  line L8781 (271.7163, 163.369) -> (271.7764, 163.3833) construction
  line L8782 (271.7764, 163.3833) -> (271.8658, 163.4071) construction
  line L8783 (271.8658, 163.4071) -> (271.9837, 163.4435) construction
  line L8784 (271.9837, 163.4435) -> (272.1293, 163.4951) construction
  line L8785 (272.1293, 163.4951) -> (272.2736, 163.5511) construction
  line L8786 (272.2736, 163.5511) -> (272.4172, 163.6099) construction
  line L8787 (272.4172, 163.6099) -> (272.5603, 163.6701) construction
  line L8788 (272.5603, 163.6701) -> (272.7031, 163.7313) construction
  line L8789 (272.7031, 163.7313) -> (272.8456, 163.7935) construction
  line L8790 (272.8456, 163.7935) -> (272.9877, 163.8571) construction
  line L8791 (272.9877, 163.8571) -> (273.1291, 163.9226) construction
  line L8792 (273.1291, 163.9226) -> (273.2699, 163.9902) construction
  line L8793 (273.2699, 163.9902) -> (273.4099, 164.06) construction
  line L8794 (273.4099, 164.06) -> (273.5493, 164.1316) construction
  line L8795 (273.5493, 164.1316) -> (273.6881, 164.205) construction
  line L8796 (273.6881, 164.205) -> (273.8264, 164.2797) construction
  line L8797 (273.8264, 164.2797) -> (273.9642, 164.3557) construction
  line L8798 (273.9642, 164.3557) -> (274.1017, 164.4327) construction
  line L8799 (274.1017, 164.4327) -> (274.2387, 164.5109) construction
  line L8800 (274.2387, 164.5109) -> (274.3752, 164.5904) construction
  line L8801 (274.3752, 164.5904) -> (274.5112, 164.6711) construction
  line L8802 (274.5112, 164.6711) -> (274.6468, 164.753) construction
  line L8803 (274.6468, 164.753) -> (274.7818, 164.8363) construction
  line L8804 (274.7818, 164.8363) -> (274.9163, 164.9208) construction
  line L8805 (274.9163, 164.9208) -> (275.0504, 165.0064) construction
  line L8806 (275.0504, 165.0064) -> (275.184, 165.0932) construction
  line L8807 (275.184, 165.0932) -> (275.3172, 165.181) construction
  line L8808 (275.3172, 165.181) -> (275.45, 165.2698) construction
  line L8809 (275.45, 165.2698) -> (275.5823, 165.3597) construction
  line L8810 (275.5823, 165.3597) -> (275.7141, 165.4506) construction
  line L8811 (275.7141, 165.4506) -> (275.8455, 165.5425) construction
  line L8812 (275.8455, 165.5425) -> (275.9765, 165.6354) construction
  line L8813 (275.9765, 165.6354) -> (276.107, 165.7293) construction
  line L8814 (276.107, 165.7293) -> (276.237, 165.8242) construction
  line L8815 (276.237, 165.8242) -> (276.3666, 165.92) construction
  line L8816 (276.3666, 165.92) -> (276.4958, 166.0168) construction
  line L8817 (276.4958, 166.0168) -> (276.6246, 166.1146) construction
  line L8818 (276.6246, 166.1146) -> (276.7529, 166.2132) construction
  line L8819 (276.7529, 166.2132) -> (276.8808, 166.3127) construction
  line L8820 (276.8808, 166.3127) -> (277.0082, 166.4131) construction
  line L8821 (277.0082, 166.4131) -> (277.1352, 166.5144) construction
  line L8822 (277.1352, 166.5144) -> (277.2618, 166.6166) construction
  line L8823 (277.2618, 166.6166) -> (277.388, 166.7196) construction
  line L8824 (277.388, 166.7196) -> (277.5137, 166.8235) construction
  line L8825 (277.5137, 166.8235) -> (277.639, 166.9283) construction
  line L8826 (277.639, 166.9283) -> (277.7638, 167.0338) construction
  line L8827 (277.7638, 167.0338) -> (277.8882, 167.1402) construction
  line L8828 (277.8882, 167.1402) -> (278.0122, 167.2474) construction
  line L8829 (278.0122, 167.2474) -> (278.1358, 167.3555) construction
  line L8830 (278.1358, 167.3555) -> (278.2589, 167.4643) construction
  line L8831 (278.2589, 167.4643) -> (278.3817, 167.5739) construction
  line L8832 (278.3817, 167.5739) -> (278.5039, 167.6842) construction
  line L8833 (278.5039, 167.6842) -> (278.6258, 167.7954) construction
  line L8834 (278.6258, 167.7954) -> (278.7472, 167.9073) construction
  line L8835 (278.7472, 167.9073) -> (278.8682, 168.02) construction
  line L8836 (278.8682, 168.02) -> (278.9888, 168.1335) construction
  line L8837 (278.9888, 168.1335) -> (279.1089, 168.2477) construction
  line L8838 (279.1089, 168.2477) -> (279.2286, 168.3626) construction
  line L8839 (279.2286, 168.3626) -> (279.3479, 168.4782) construction
  line L8840 (279.3479, 168.4782) -> (279.4667, 168.5946) construction
  line L8841 (279.4667, 168.5946) -> (279.5851, 168.7118) construction
  line L8842 (279.5851, 168.7118) -> (279.7031, 168.8296) construction
  line L8843 (279.7031, 168.8296) -> (279.8207, 168.9481) construction
  line L8844 (279.8207, 168.9481) -> (279.9378, 169.0674) construction
  line L8845 (279.9378, 169.0674) -> (280.0545, 169.1873) construction
  line L8846 (280.0545, 169.1873) -> (280.1708, 169.3079) construction
  line L8847 (280.1708, 169.3079) -> (280.2866, 169.4293) construction
  line L8848 (280.2866, 169.4293) -> (280.402, 169.5512) construction
  line L8849 (280.402, 169.5512) -> (280.517, 169.6739) construction
  line L8850 (280.517, 169.6739) -> (280.6087, 169.7726) construction
  line L8851 (280.6087, 169.7726) -> (280.6772, 169.8469) construction
  line L8852 (280.6772, 169.8469) -> (280.7228, 169.8966) construction
  line L8853 (280.7228, 169.8966) -> (280.7456, 169.9215) construction
  spline S118 degree 5 poles (236.3268, 93.9655) (236.3391, 93.9372) (236.3628, 93.8802) (236.396, 93.7938) (236.4359, 93.6771) (236.4798, 93.5289) (236.5193, 93.3792) (236.5561, 93.2286) (236.5915, 93.0774) (236.626, 92.9259) (236.6594, 92.774) (236.6914, 92.6217) (236.7216, 92.4688) (236.7496, 92.3152) (236.7755, 92.1609) (236.7994, 92.006) (236.8217, 91.8506) (236.8425, 91.6948) (236.8621, 91.5386) (236.8805, 91.3821) (236.8978, 91.2253) (236.9138, 91.0682) (236.9285, 90.9107) (236.9418, 90.7529) (236.9538, 90.5947) (236.9645, 90.4362) (236.974, 90.2774) (236.9824, 90.1183) (236.9897, 89.9589) (236.9958, 89.7993) (237.0009, 89.6395) (237.0049, 89.4794) (237.0077, 89.3191) (237.0096, 89.1585) (237.0103, 88.9977) (237.01, 88.8367) (237.0086, 88.6755) (237.0062, 88.5141) (237.0028, 88.3525) (236.9985, 88.1907) (236.9931, 88.0288) (236.9868, 87.8666) (236.9795, 87.7043) (236.9712, 87.5419) (236.962, 87.3793) (236.9519, 87.2165) (236.9408, 87.0536) (236.9287, 86.8905) (236.9158, 86.7273) (236.902, 86.564) (236.8872, 86.4005) (236.8716, 86.2369) (236.855, 86.0732) (236.8376, 85.9094) (236.8193, 85.7455) (236.8001, 85.5815) (236.78, 85.4174) (236.7591, 85.2532) (236.7374, 85.0889) (236.7148, 84.9245) (236.6913, 84.76) (236.667, 84.5954) (236.6418, 84.4308) (236.6159, 84.266) (236.5891, 84.1013) (236.5614, 83.9364) (236.533, 83.7715) (236.5038, 83.6065) (236.4737, 83.4415) (236.4428, 83.2764) (236.4112, 83.1113) (236.3852, 82.9792) (236.3654, 82.8801) (236.352, 82.814) (236.3452, 82.7809) knots 0 0 0 0 0 0 0.01428571 0.02857143 0.04285714 0.05714286 0.07142857 0.08571429 0.1 0.11428571 0.12857143 0.14285714 0.15714286 0.17142857 0.18571429 0.2 0.21428571 0.22857143 0.24285714 0.25714286 0.27142857 0.28571429 0.3 0.31428571 0.32857143 0.34285714 0.35714286 0.37142857 0.38571429 0.4 0.41428571 0.42857143 0.44285714 0.45714286 0.47142857 0.48571429 0.5 0.51428571 0.52857143 0.54285714 0.55714286 0.57142857 0.58571429 0.6 0.61428571 0.62857143 0.64285714 0.65714286 0.67142857 0.68571429 0.7 0.71428571 0.72857143 0.74285714 0.75714286 0.77142857 0.78571429 0.8 0.81428571 0.82857143 0.84285714 0.85714286 0.87142857 0.88571429 0.9 0.91428571 0.92857143 0.94285714 0.95714286 0.97142857 0.98571429 1 1 1 1 1 1
  line L8854 (236.3268, 93.9655) -> (236.3391, 93.9372) construction
  line L8855 (236.3391, 93.9372) -> (236.3628, 93.8802) construction
  line L8856 (236.3628, 93.8802) -> (236.396, 93.7938) construction
  line L8857 (236.396, 93.7938) -> (236.4359, 93.6771) construction
  line L8858 (236.4359, 93.6771) -> (236.4798, 93.5289) construction
  line L8859 (236.4798, 93.5289) -> (236.5193, 93.3792) construction
  line L8860 (236.5193, 93.3792) -> (236.5561, 93.2286) construction
  line L8861 (236.5561, 93.2286) -> (236.5915, 93.0774) construction
  line L8862 (236.5915, 93.0774) -> (236.626, 92.9259) construction
  line L8863 (236.626, 92.9259) -> (236.6594, 92.774) construction
  line L8864 (236.6594, 92.774) -> (236.6914, 92.6217) construction
  line L8865 (236.6914, 92.6217) -> (236.7216, 92.4688) construction
  line L8866 (236.7216, 92.4688) -> (236.7496, 92.3152) construction
  line L8867 (236.7496, 92.3152) -> (236.7755, 92.1609) construction
  line L8868 (236.7755, 92.1609) -> (236.7994, 92.006) construction
  line L8869 (236.7994, 92.006) -> (236.8217, 91.8506) construction